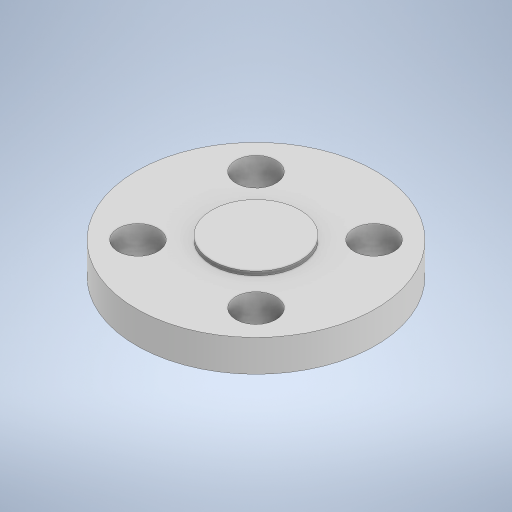
# Autodesk Inventor part: ANSI-B300-0.5B
Saved by Autodesk Inventor 2023 (Build 270158000, 158)
## iProperties
Created: 2023-11-03
Part Number: ANSI-B300-0.5B
Material: Generic
Document SubType Name: Modeling
Designer: Admin
Density: 1 g/cm^3
Appearance: Default
Author: Admin
Autodesk Inventor part; units mm, degrees
ref_plane "YZ Plane" through (0, 0, 0) normal (1, 0, 0) x (0, 1, 0)
ref_plane "XZ Plane" through (0, 0, 0) normal (0, 1, 0) x (-1, 0, 0)
ref_plane "XY Plane" through (0, 0, 0) normal (0, 0, 1) x (1, 0, 0)
sketch "Sketch1" plane through (0, 0, 0) normal (0, 0, 1) x (1, 0, 0)
  line L0 (0, 0) -> (0, 14.2875)
  line L1 (-11.176, 0) -> (-17.526, 0)
  line L2 (0, 0) -> (-47.625, 0)
  line L3 (-47.625, 0) -> (-47.625, 12.7)
  line L4 (-47.625, 12.7) -> (-17.526, 12.7)
  line L5 (-33.274, 12.7) -> (-33.274, 0) construction
  line L6 (0, 14.2875) -> (-17.526, 14.2875)
  line L7 (-17.526, 14.2875) -> (-17.526, 12.7)
  dimension "Thickness" = 12.7
  dimension "OD" = 95.25
  dimension "BC" = 66.548
  dimension "R" = 35.052
  dimension "d24" = 1.5875
  constraints: 16 end point, 4 horizontal, 4 vertical, 2 point on line, 1 horizontal alignment
  measures "Thickness" distance of L2.end L3.end
  measures "OD" diameter of L3 L0
  measures "BC" diameter of L5 L0
  measures "R" diameter of L7 L0
  measures "d24" distance between parallel lines of L6 L4
revolve "Revolution1" add sketch "Sketch1" angle 360 about axis through (0, 0, 0) along (0, 1, 0)
sketch "Sketch2" plane through (0, 12.7, 0) normal (0, 1, 0) x (1, 0, 0)
  line L0 (0, 0) -> (0, 47.625) construction
  circle A0 centre (0, 0) radius 47.625 projected
  line L1 (0, 0) -> (23.5283, 23.5283) construction
  dimension "d11" = 45
  dimension "d12" = 33.274
  constraints: 4 end point, 1 coincident, 1 vertical, 1 vertical alignment, 1 other
  measures "d11" angle of L1 L0
  measures "d12" distance of L1.start L1.end
hole "Hole1" at (23.5283, 12.7, -23.5283) direction (0, -1, 0) diameter 16.002 depth 12.7
pattern_circular "Circular Pattern1" count 4 over 360 about axis through (0, -10, 0) along (0, 1, 0) of "Hole1"
equation "\"d12\" = 0.5 * BC"
body "Solid1"
